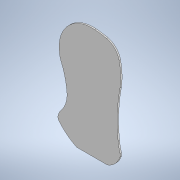
# Autodesk Inventor part: Grundform_Nao_Schuh_original
Saved by Autodesk Inventor 2020 (Build 240168000, 168)
## iProperties
Created: 2020-02-10
Part Number: Grundform_Nao_Schuh_original
Material: Generic
Document SubType Name: Modeling
Designer: Mara
Density: 1 g/cm^3
Appearance: Default
Author: Mara
## iProperties of the stored document _3DPrint.ipt
Created: 2020-02-11
Part Number: _3DPrint
Material: Generic
Document SubType Name: Modeling
Designer: Mara
Density: 1 g/cm^3
Appearance: Default
Author: Mara
Autodesk Inventor part; units mm, degrees
ref_plane "YZ Plane" through (0, 0, 0) normal (1, 0, 0) x (0, 1, 0)
ref_plane "XZ Plane" through (0, 0, 0) normal (0, 1, 0) x (-1, 0, 0)
ref_plane "XY Plane" through (0, 0, 0) normal (0, 0, 1) x (1, 0, 0)
sketch "Sketch1" plane through (0, 0, 0) normal (0, 0, 1) x (1, 0, 0)
  arc A0 (17, 50.9482) -> (0, 53.5) centre (-5.1444, -38.6736) ccw
  arc A1 (34.618, 33) -> (17, 50.9482) centre (11.2519, 27.6848) ccw
  arc A2 (36, 0) -> (34.618, 33) centre (-54.4409, 12.7413) ccw
  line L0 (36, 0) -> (36, -81) construction
  arc A3 (-50, 0) -> (-47.876, -9) centre (-23.2557, 1.561) ccw
  line L1 (-50, 0) -> (-52.0013, -78) construction
  arc A4 (-39.1762, -46) -> (-47.876, -9) centre (-148.6013, -52.2064) ccw
  arc A5 (-48.0013, -70.0072) -> (-39.1762, -46) centre (-76.244, -45.9995) ccw
  arc A6 (-48.0013, -70.0072) -> (-52.0013, -78) centre (-33.7069, -82.1582) ccw
  line L2 (36, 0) -> (36, -81) construction
  arc A7 (0, 53.5) -> (-50, 0) centre (-4.0952, 7.2128) ccw
  arc A8 (-52.0013, -78) -> (-50.4909, -84.4368) centre (-45.2921, -79.8213) ccw
  arc A9 (-50.4909, -84.4368) -> (-25.5013, -104) centre (5.8002, -38.274) ccw
  line L3 (-25.5013, -104) -> (18, -104)
  arc A10 (36, 0) -> (33.2377, -67.2753) centre (254.1506, -42.6516) ccw
  arc A11 (18, -104) -> (35.9231, -85.173) centre (7.7888, -76.3343) ccw
  arc A12 (33.2377, -67.2753) -> (36, -81) centre (112.7493, -58.4127) ccw
  arc A13 (35.9231, -85.173) -> (36, -81) centre (29.326, -82.9642) ccw
  point P0 (0, 0)
  dimension "d6" = 53.5
  dimension "d7" = 50
  dimension "d8" = 36
  dimension "d10" = 81
  dimension "d16" = 78
  dimension "d18" = 9
  dimension "d24" = 4
  dimension "d28" = 33
  dimension "d29" = 46
  dimension "d33" = 104
  dimension "d34" = 26.5
  dimension "d35" = 18
  dimension "d36" = 0
  dimension "d38" = 92.317
  dimension "d39" = 91.334
  dimension "d40" = 46.468
  dimension "d41" = 26.7899
  dimension "d42" = 222.281
  dimension "d43" = 80.004
  dimension "d44" = 109.601
  dimension "d45" = 37.0678
  dimension "d46" = 18.761
  dimension "d47" = 6.952
  dimension "d48" = 72.799
  dimension "d49" = 29.49
  dimension "d50" = 6.957
  dimension "d51" = 17
  dimension "d52" = 0
  dimension "d53" = 23.963
  dimension "d54" = 50
  dimension "d55" = 2.0013
  dimension "d56" = 12.0001
  dimension "d57" = 67.2753
  dimension "d58" = 18.827
  dimension "d59" = 19.5632
  dimension "d61" = 24.9896
  constraints: 28 point on circle, 14 centre point, 9 end point, 6 tangent, 1 collinear, 1 horizontal, 1 vertical
  measures "d6" distance of point (0, 0) A0.end
  measures "d7" distance of point (0, 0) L1.start
  measures "d8" distance of L0.start point (0, 0)
  measures "d10" distance of L0.start L0.end
  measures "d16" vertical distance of L1.start L1.end
  measures "d18" vertical distance of L1.start A3.end
  measures "d24" horizontal distance of L1.end A5.start
  measures "d28" vertical distance of point (0, 0) A1.start
  measures "d29" vertical distance of A4.start point (0, 0)
  measures "d33" distance from line of L3 point (0, 0)
  measures "d34" horizontal distance of L1.end L3.start
  measures "d35" horizontal distance of L3.end L0.end
  measures "d36" vertical distance of L0.start point (0, 0)
  measures "d38" radius of A0
  measures "d39" radius of A2
  measures "d40" radius of A7
  measures "d41" radius of A3
  measures "d42" radius of A10
  measures "d43" radius of A12
  measures "d44" radius of A4
  measures "d45" radius of A5
  measures "d46" radius of A6
  measures "d47" radius of A8
  measures "d48" radius of A9
  measures "d49" radius of A11
  measures "d50" radius of A13
  measures "d51" horizontal distance of A0.end A0.start
  measures "d52" horizontal distance of point (0, 0) A0.end
  measures "d53" radius of A1
  measures "d54" distance of point (0, 0) L1.start
  measures "d55" horizontal distance of L1.start L1.end
  measures "d56" distance from line of L1 A4.start
  measures "d57" vertical distance of L0.start A10.end
  measures "d58" vertical distance of L3.end A11.end
  measures "d59" vertical distance of A8.end L3.start
  measures "d61" horizontal distance of L3.start A8.end
extrude "Extrusion1" add sketch "Sketch1" along normal blind 2
body "Solid1"
